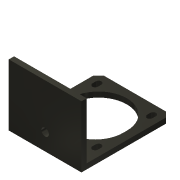
# Autodesk Inventor part: StepperMount
Saved by Autodesk Inventor 2014 (Build 180170000, 170)
## iProperties
Created: 2014-08-10
Part Number: StepperMount
Material: Generic
Document SubType Name: Modeling
Designer: Peele
Density: 1 g/cm^3
Appearance: Gunmetal
Author: Peele
Autodesk Inventor part; units mm, degrees
ref_plane "YZ Plane" through (0, 0, 0) normal (1, 0, 0) x (0, 1, 0)
ref_plane "XZ Plane" through (0, 0, 0) normal (0, 1, 0) x (-1, 0, 0)
ref_plane "XY Plane" through (0, 0, 0) normal (0, 0, 1) x (1, 0, 0)
sketch "Sketch1" plane through (0, 0, 0) normal (0, 0, 1) x (1, 0, 0)
  line L0 (-20.65, -25.5) -> (20.65, -25.5)
  line L1 (20.65, -25.5) -> (20.65, 25.5)
  line L2 (20.65, 25.5) -> (-20.65, 25.5)
  line L3 (-20.65, 25.5) -> (-20.65, -25.5)
  line L4 (-20.65, -25.5) -> (20.65, 25.5) construction
  line L5 (20.65, -25.5) -> (-20.65, 25.5) construction
  line L6 (0, 2.9) -> (0, 4.9) construction
  line L7 (16, 2.9) -> (16, 4.9)
  line L8 (-16, 4.9) -> (-16, 2.9)
  arc A0 (-16, 2.9) -> (16, 2.9) centre (0, 2.9) ccw
  arc A1 (16, 4.9) -> (-16, 4.9) centre (0, 4.9) ccw
  line L9 (-15.5, 20.4) -> (-15.5, 18.4) construction
  line L10 (-17.1, 20.4) -> (-17.1, 18.4)
  line L11 (-13.9, 18.4) -> (-13.9, 20.4)
  arc A2 (-13.9, 20.4) -> (-17.1, 20.4) centre (-15.5, 20.4) ccw
  arc A3 (-17.1, 18.4) -> (-13.9, 18.4) centre (-15.5, 18.4) ccw
  line L12 (15.5, 20.4) -> (15.5, 18.4) construction
  line L13 (13.9, 20.4) -> (13.9, 18.4)
  line L14 (17.1, 18.4) -> (17.1, 20.4)
  arc A4 (17.1, 20.4) -> (13.9, 20.4) centre (15.5, 20.4) ccw
  arc A5 (13.9, 18.4) -> (17.1, 18.4) centre (15.5, 18.4) ccw
  line L15 (15.5, -10.6) -> (15.5, -12.6) construction
  line L16 (13.9, -10.6) -> (13.9, -12.6)
  line L17 (17.1, -12.6) -> (17.1, -10.6)
  arc A6 (17.1, -10.6) -> (13.9, -10.6) centre (15.5, -10.6) ccw
  arc A7 (13.9, -12.6) -> (17.1, -12.6) centre (15.5, -12.6) ccw
  line L18 (-15.5, -10.6) -> (-15.5, -12.6) construction
  line L19 (-17.1, -10.6) -> (-17.1, -12.6)
  line L20 (-13.9, -12.6) -> (-13.9, -10.6)
  arc A8 (-13.9, -10.6) -> (-17.1, -10.6) centre (-15.5, -10.6) ccw
  arc A9 (-17.1, -12.6) -> (-13.9, -12.6) centre (-15.5, -12.6) ccw
  point P0 (0, 0)
  point P1 (0, 3.9)
  point P2 (-15.5, 19.4)
  point P3 (15.5, 19.4)
  point P4 (15.5, -11.6)
  point P5 (-15.5, -11.6)
  dimension "d0" = 51
  dimension "d1" = 41.3
  dimension "d2" = 28.4
  dimension "d3" = 2
  dimension "d4" = 16
  dimension "d5" = 2
  dimension "d6" = 31
  dimension "d7" = 31
  dimension "d8" = 1.6
  dimension "d10" = 15.5
  dimension "d11" = 15.5
  constraints: 52 end point, 20 point on circle, 20 tangent, 12 parallel, 10 centre point, 7 midpoint, 3 equal length, 3 equal radius, 2 collinear, 2 horizontal alignment, 1 horizontal, 1 perpendicular, 1 vertical alignment
  measures "d0" distance of L2.end L0.start
  measures "d1" distance of L1.end L2.end
  measures "d2" distance from line of L6.start L0
  measures "d3" distance of L6.start L6.end
  measures "d4" radius of A1
  measures "d5" distance of L9.start L9.end
  measures "d6" distance of L18.start L9.start
  measures "d7" distance of L12.start L9.start
  measures "d8" radius of A2
  measures "d10" distance from line of point (0, 0) L9
  measures "d11" horizontal distance of point (0, 3.9) point (-15.5, 19.4)
extrude "Extrusion1" add sketch "Sketch1" along normal blind 3
sketch "Sketch2" plane through (-20.65, -25.5, 0) normal (0, -1, 0) x (1, 0, 0)
  line L0 (0, 0) -> (41.3, 0) projected
  line L1 (41.3, 0) -> (41.3, 3) projected
  line L2 (0, 0) -> (41.3, 0)
  line L3 (41.3, 0) -> (41.3, 35)
  line L4 (41.3, 35) -> (0, 35)
  line L5 (0, 35) -> (0, 0)
  circle A0 centre (20.65, 9.5) radius 2.15
  point P0 (20.65, 0)
  dimension "d14" = 35
  dimension "d15" = 9.5
  dimension "d16" = 4.3
  constraints: 8 end point, 2 parallel, 1 centre point, 1 collinear, 1 horizontal, 1 perpendicular
  measures "d14" distance of L4.end L0.start
  measures "d15" distance from line of A0.centre L0
  measures "d16" diameter of A0
extrude "Extrusion2" add sketch "Sketch2" against normal blind 3
chamfer "Chamfer1" distance 3 angle 45 2 edges at (20.65, 25.5, 1.5) (-20.65, 25.5, 1.5)
equation "\"d10\" = 0.5 * d7"
equation "\"d11\" = 0.5 * d6"
body "Solid1"
